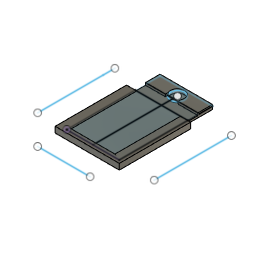
2022_09_12_MagnetsMidiJackHolder v2 (Autodesk Fusion 360 design; units mm, degrees)
Autodesk Fusion 360 part; units mm, degrees
sketch "Sketch1" plane through (0, 0, 0) normal (0, 0, 1) x (1, 0, 0)
  line L0 (0, 0) -> (18, 0)
  line L1 (18, 0) -> (18, 23.5)
  line L2 (0, 0) -> (18, 0)
  line L3 (18, 0) -> (18, 23.5)
  line L4 (18, 23.5) -> (0, 23.5)
  line L5 (0, 23.5) -> (0, 0)
  line L6 (9, 0) -> (9, 27.5)
  line L7 (9, 27.5) -> (18, 27.5)
  line L8 (18, 27.5) -> (18, 31.9976)
  line L9 (18, 31.9976) -> (0, 31.9976)
  line L10 (0, 31.9976) -> (0, 27.5)
  line L11 (0, 27.5) -> (9, 27.5)
  line L12 (18, 23.5) -> (18, 31.9976) construction
  dimension "d1" = 18
  dimension "d2" = 23.5
  dimension "d11" = 27.5
  constraint coincident L0.start L2.start
  constraint horizontal L0
  constraint perpendicular L0 L1
  constraint horizontal L2
  constraint vertical L3
  constraint horizontal L4
  constraint vertical L5
  constraint midpoint L2 L6.start
  constraint perpendicular L4 L6
  constraint perpendicular L6 L7
  constraint perpendicular L7 L8
  constraint perpendicular L6 L9
  constraint perpendicular L9 L10
  constraint perpendicular L6 L11
  constraint perpendicular L4 L12
  constraint coincident L8.end L9.start
  measures "d1" distance of L0.start L0.end
  measures "d2" distance of L0.end L1.end
  measures "d11" distance of L6.start L6.end
sketch "Sketch2" plane through (0, 0, 0) normal (0, 1, 0) x (1, 0, 0)
  line L0 (0, 0) -> (18, 0)
  line L1 (18, 0) -> (16.5, -1.0004)
  line L2 (0, 0) -> (1.5, -1.0004)
  line L3 (0, 0) -> (5, 0) construction
  line L4 (1.5, -1.0004) -> (-1, -1.0004)
  line L5 (-1, -1.0004) -> (-1, 1)
  line L6 (-1, 1) -> (19.0195, 1)
  line L7 (19.0195, 1) -> (19.0195, -1.0004)
  line L8 (19.0195, -1.0004) -> (16.5, -1.0004)
  line L9 (1.5, -1.0004) -> (16.5, -1.0004)
  dimension "d3" = 33.7
  dimension "d4" = 33.7
  dimension "d6" = 1.803
  dimension "d27" = 18
  dimension "d31" = 1.803
  constraint coincident L0.start L2.start
  constraint horizontal L0
  constraint horizontal L3
  constraint horizontal L4
  constraint perpendicular L4 L5
  constraint perpendicular L5 L6
  constraint perpendicular L6 L7
  constraint perpendicular L7 L8
  measures "d3" angle of L0 L1
  measures "d4" angle of L2 L3
  measures "d6" distance of L0.end L1.end
  measures "d27" distance of L0.start L0.end
  measures "d31" distance of L0.start L2.end
extrude "Extrude1" add sketch "Sketch2" along normal blind 22.5 contours L0 L1 L2 L4 L5 L6 L7 L8 makes body 1
extrude "Extrude2" add sketch "Sketch2" against normal blind 2 bodies 1
extrude "Extrude3" add sketch "Sketch1" against normal blind 1 separate body contours L7 L8 L9 L10 L11 makes body 2
extrude "Extrude4" add 2 faces at (3, 27.5, -0.3333) (12, 27.5, -0.3333) along direction (0, -1, 0) blind 5 on bodies 2 bodies 2 1
extrude "Extrude5" add sketch "Sketch1" along normal blind 0.2 contours L7 L8 L9 L10 L11 bodies 2
sketch "Sketch3" plane through (0, 0, 0) normal (0, 0, 1) x (-1, 0, 0)
  line L0 (-18, -27.5) -> (0, -27.5)
  line L1 (0, -27.5) -> (0, -22.5)
  line L2 (0, -22.5) -> (0, 0)
  line L3 (-18, 0) -> (-18, -22.5)
  line L4 (-18, -22.5) -> (-18, -27.5)
  circle A0 centre (-9, -29) radius 2.3776
  line L5 (0, 0) -> (-18, 0)
extrude "Extrude6" cut sketch "Sketch3" against normal blind 0.8 contours L0 A0 | L0 A0 bodies 2
extrude "Extrude7" cut sketch "Sketch3" along normal blind 1.5 contours L0 A0 | L0 A0 bodies 2
extrude "Extrude8" cut sketch "Sketch3" sketch "Sketch1" against normal blind 0.3 contours L0 L1 L2 L3 L4 A0 L5 of sketch 2 contours L0 L2 L4 L5 L6 bodies 2
extrude "Extrude9" add 1 faces at (2.216, 29.6154, 0.2) along direction (0, 0, 1) blind 0.3 on bodies 2 bodies 2
extrude "Extrude10" cut 2 faces at (15.6149, 27.5, -0.0333) (2.3851, 27.5, 0.2333) along direction (0, 1, 0) blind 0.5 on bodies 2 bodies 2
sketch "Sketch4" plane through (0, 0, 0) normal (0, 0, 1) x (1, 0, 0)
  line L0 (0, -10) -> (18, -10)
  line L1 (30, 0) -> (30, 26.5)
  line L2 (-10, 0) -> (-10, 22.5)
  line L3 (-10, 22.5) -> (-10, 26.5)
  dimension "d32" = 18
  dimension "d34" = 26.5
  dimension "d35" = 22.5
  dimension "d36" = 4
  constraint horizontal L0
  constraint vertical L1
  constraint vertical L2
  constraint parallel L2 L3
  measures "d32" distance of L0.start L0.end
  measures "d34" distance of L1.start L1.end
  measures "d35" distance of L2.start L2.end
  measures "d36" distance of L2.end L3.end
extrude "Extrude11" add 2 faces at (4.5619, 28, 0.2333) (13.4381, 28, 0.2333) along direction (0, -1, 0) blind 1 on bodies 2 bodies 2
extrude "Extrude12" add 1 faces at (-1, 6.1667, 0.3336) along direction (-1, 0, 0) blind 1 on bodies 2 bodies 2
extrude "Extrude13" add 1 faces at (19.0195, 6.1667, -0.3332) along direction (1, 0, 0) blind 1 on bodies 2 bodies 2
equation "d36 = 26.5 mm - 22.5 mm"
